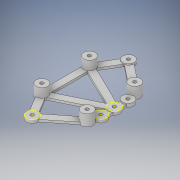
# Autodesk Inventor part: mount
Saved by Autodesk Inventor 2019 (Build 230136000, 136)
## iProperties
Created: 2019-01-14
Part Number: mount
Material: Generic
Document SubType Name: Modeling
Designer: erwin
Density: 1 g/cm^3
Appearance: Default
Author: erwin
Autodesk Inventor part; units mm, degrees
ref_plane "YZ Plane" through (0, 0, 0) normal (1, 0, 0) x (0, 1, 0)
ref_plane "XZ Plane" through (0, 0, 0) normal (0, 1, 0) x (-1, 0, 0)
ref_plane "XY Plane" through (0, 0, 0) normal (0, 0, 1) x (1, 0, 0)
sketch "Sketch1" plane through (0, 0, 0) normal (0, 1, 0) x (-1, 0, 0)
  point P0 (0, 0)
  point P1 (0, 0)
  point P2 (0, -12)
  point P3 (0, 12)
  point P4 (30, -42.5)
  point P5 (30, 42.5)
  dimension "d0" = 85
  dimension "d1" = 12
  dimension "d2" = 12
  dimension "d3" = 30
  dimension "d4" = 30.5
  dimension "d5" = 30.5
  constraints: 1 coincident
  measures "d0" distance of point (30, -42.5) point (30, 42.5)
  measures "d1" distance of point (0, 0) point (0, 12)
  measures "d2" distance of point (0, -12) point (0, 0)
  measures "d3" horizontal distance of point (30, 42.5) point (0, 12)
  measures "d4" vertical distance of point (0, 12) point (30, 42.5)
  measures "d5" vertical distance of point (0, -12) point (30, -42.5)
sketch "Sketch2" plane through (0, 0, 0) normal (0, 1, 0) x (-1, 0, 0)
  circle A0 centre (30, 42.5) radius 5
  point P0 (0, 0)
  dimension "d6" = 10
  constraints: 1 centre point, 1 coincident
  measures "d6" diameter of A0
extrude "Extrusion1" add sketch "Sketch2" along normal blind 3
sketch "Sketch3" plane through (-30, 3, 42.5) normal (0, 1, 0) x (1, 0, 0)
  circle A0 centre (0, 0) radius 5 projected
  point P0 (30, 42.5)
hole "Hole1" at (-30, 3, 42.5) direction (0, -1, 0) diameter 3 end through all both
pattern_sketch "Sketch Driven Pattern1" of "Extrusion1", "Hole1" from (-30, 0, 42.5) copies at (0, 0, 0) at (0, 0, -12) at (0, 0, 12) at (-30, 0, -42.5)
sketch "Sketch4" plane through (-30, 3, 42.5) normal (0, 1, 0) x (1, 0, 0)
  circle A0 centre (0, 0) radius 5 projected
  circle A1 centre (30, 30.5) radius 5 projected
  circle A2 centre (30, 42.5) radius 5 projected
  point P0 (30, 42.5)
sketch "Sketch5" plane through (0, 0, -12) normal (0, -1, 0) x (1, 0, 0)
  line L0 (-43, 33) -> (-3, 33) construction
  line L1 (-3, 33) -> (-3, -9) construction
  line L2 (-3, -9) -> (-43, -9) construction
  line L3 (-43, -9) -> (-43, 33) construction
  circle A0 centre (-30, 54.5) radius 1.5 construction
  circle A1 centre (-30, -30.5) radius 1.5 construction
  circle A2 centre (-43, 33) radius 5
  circle A3 centre (-43, -9) radius 5
  circle A4 centre (-3, -9) radius 5
  circle A5 centre (-3, 33) radius 5
  point P0 (0, 12)
  dimension "d16" = 40
  dimension "d17" = 42
  dimension "d18" = 3
  dimension "d19" = 21.5
  dimension "d20" = 21.5
  dimension "d21" = 10
  dimension "d22" = 10
  dimension "d23" = 10
  dimension "d24" = 10
  constraints: 8 end point, 4 centre point, 4 coincident, 2 parallel, 1 horizontal, 1 perpendicular
  measures "d16" distance of L1.end L2.end
  measures "d17" distance of L0.end L1.end
  measures "d18" distance from line of point (0, 12) L1
  measures "d19" distance from line of A0.centre L0
  measures "d20" distance from line of L2 A1.centre
  measures "d21" diameter of A2
  measures "d22" diameter of A3
  measures "d23" diameter of A4
  measures "d24" diameter of A5
extrude "Extrusion2" add sketch "Sketch5" against normal blind 10
sketch "Sketch7" plane through (-43, 10, 21) normal (0, 1, 0) x (1, 0, 0)
  circle A0 centre (0, 0) radius 5 projected
  circle A1 centre (0, 42) radius 5 projected
  circle A2 centre (40, 0) radius 5 projected
  circle A3 centre (40, 42) radius 5 projected
  point P0 (43, 21)
  constraints: 4 coincident
hole "Hole2" at (-43, 10, 21) at (-43, 10, -21) at (-3, 10, 21) at (-3, 10, -21) direction (0, -1, 0) diameter 3 end through all both
sketch "Sketch8" plane through (-30, 0, 42.5) normal (0, -1, 0) x (1, 0, 0)
  circle A0 centre (-13, -21.5) radius 1.5 projected
  circle A1 centre (-13, -21.5) radius 5 projected
  circle A2 centre (-13, -63.5) radius 1.5 projected
  circle A3 centre (-13, -63.5) radius 5 projected
  circle A4 centre (0, -85) radius 1.5 projected
  circle A5 centre (0, -85) radius 5 projected
  circle A6 centre (27, -21.5) radius 1.5 projected
  arc A7 (30, -25.5) -> (27, -26.5) centre (27, -21.5) ccw projected
  arc A8 (27, -26.5) -> (30, -25.5) centre (30, -30.5) ccw projected
  circle A9 centre (30, -30.5) radius 1.5 projected
  circle A10 centre (27, -63.5) radius 1.5 projected
  arc A11 (27, -58.5) -> (30, -59.5) centre (27, -63.5) ccw projected
  arc A12 (30, -59.5) -> (27, -58.5) centre (30, -54.5) ccw projected
  circle A13 centre (30, -54.5) radius 1.5 projected
  circle A14 centre (30, -42.5) radius 1.5 projected
  circle A15 centre (30, -42.5) radius 5 projected
  circle A16 centre (0, 0) radius 1.5 projected
  circle A17 centre (0, 0) radius 5 projected
  line L0 (0, 0) -> (-13, -21.5)
  line L1 (-13, -21.5) -> (-13, -63.5)
  line L2 (-13, -63.5) -> (0, -85)
  line L3 (0, -85) -> (27, -63.5)
  line L4 (0, 0) -> (27, -21.5)
  line L5 (30, -30.5) -> (30, -42.5)
  line L6 (30, -54.5) -> (30, -42.5)
  line L7 (0, 0) -> (-13, -21.5) construction
  line L8 (-4.6369, -1.8707) -> (-13.4975, -16.5248)
  arc A18 (2.5672, -1.5523) -> (-2.5672, 1.5523) centre (0, 0) ccw
  arc A19 (-15.5672, -19.9477) -> (-10.4328, -23.0523) centre (-13, -21.5) ccw
  line L9 (-13, -21.5) -> (-13, -63.5) construction
  line L10 (-16, -25.5) -> (-16, -59.5)
  arc A20 (-10, -21.5) -> (-16, -21.5) centre (-13, -21.5) ccw
  arc A21 (-16, -63.5) -> (-10, -63.5) centre (-13, -63.5) ccw
  line L11 (-13, -63.5) -> (0, -85) construction
  line L12 (-13.4975, -68.4752) -> (-4.6369, -83.1293)
  arc A22 (-10.4328, -61.9477) -> (-15.5672, -65.0523) centre (-13, -63.5) ccw
  arc A23 (-2.5672, -86.5523) -> (2.5672, -83.4477) centre (0, -85) ccw
  line L13 (0, -85) -> (27, -63.5) construction
  line L14 (4.9979, -84.8551) -> (25.7397, -68.3385)
  arc A24 (-1.8688, -82.6532) -> (1.8688, -87.3468) centre (0, -85) ccw
  arc A25 (28.8688, -65.8468) -> (25.1312, -61.1532) centre (27, -63.5) ccw
  line L15 (0, 0) -> (27, -21.5) construction
  line L16 (25.7397, -16.6615) -> (4.9979, -0.1449)
  arc A26 (1.8688, 2.3468) -> (-1.8688, -2.3468) centre (0, 0) ccw
  arc A27 (25.1312, -23.8468) -> (28.8688, -19.1532) centre (27, -21.5) ccw
  line L17 (30, -30.5) -> (30, -54.5) construction
  arc A28 (33, -30.5) -> (27, -30.5) centre (30, -30.5) ccw
  arc A29 (27, -54.5) -> (33, -54.5) centre (30, -54.5) ccw
  line L18 (33, -50.5) -> (33, -46.5)
  line L19 (33, -38.5) -> (33, -34.5)
  line L20 (27, -34.5) -> (27, -38.5)
  line L21 (27, -46.5) -> (27, -50.5)
  line L22 (22.0021, -63.6449) -> (1.2603, -80.1615)
  line L23 (-1.5652, -82.4114) -> (-1.8688, -82.6532)
  line L24 (2.5672, -83.4477) -> (2.3664, -83.1156)
  line L25 (0.4975, -80.0248) -> (-8.3631, -65.3707)
  line L26 (-10, -62.6635) -> (-10.4328, -61.9477)
  line L27 (-10, -63.5) -> (-10, -62.6635)
  line L28 (-10, -59.5) -> (-10, -25.5)
  line L29 (-10, -22.3365) -> (-10, -21.5)
  line L30 (-10.4328, -23.0523) -> (-10, -22.3365)
  line L31 (-8.3631, -19.6293) -> (0.4975, -4.9752)
  line L32 (2.3664, -1.8844) -> (2.5672, -1.5523)
  line L33 (-1.8688, -2.3468) -> (-1.5652, -2.5886)
  line L34 (1.2603, -4.8385) -> (22.0021, -21.3551)
  point P0 (30, -42.5)
  point P1 (-6.5, -10.75)
  point P2 (-13, -42.5)
  point P3 (-6.5, -74.25)
  point P4 (13.5, -74.25)
  point P5 (13.5, -10.75)
  dimension "d34" = 6
  dimension "d35" = 6
  dimension "d36" = 6
  dimension "d37" = 6
  dimension "d38" = 6
  dimension "d39" = 6
  constraints: 82 end point, 52 point on circle, 44 tangent, 20 parallel, 12 centre point, 6 midpoint, 4 collinear, 4 point on line, 3 vertical
  measures "d34" diameter of A19
  measures "d35" diameter of A21
  measures "d36" diameter of A23
  measures "d37" diameter of A25
  measures "d38" diameter of A27
  measures "d39" diameter of A29
extrude "Extrusion3" add sketch "Sketch8" against normal blind 2 contours L0 A17 L31 A1 | A1 L8 A17 L0 | L1 A3 L10 A1 | A1 L28 A3 L1 | A17 L4 A7 L34 | A3 L2 A5 L12 | A17 L16 A7 L4 | A3 L25 A5 L2 | A8 L5 A15 L20 | A5 L3 A11 L14 | L22 A11 L3 A5 | A8 L19 A15 L5 | A15 L6 A12 L21 | A15 L18 A12 L6
sketch "Sketch9" plane through (0, 0, 0) normal (0, -1, 0) x (1, 0, 0)
  circle A0 centre (0, 0) radius 1.5 projected
  circle A1 centre (-3, -21) radius 1.5 projected
  circle A2 centre (0, -12) radius 1.5 projected
  circle A3 centre (-30, 42.5) radius 1.5 projected
  circle A4 centre (-3, 21) radius 1.5 projected
  circle A5 centre (0, 12) radius 1.5 projected
  circle A6 centre (-30, -42.5) radius 1.5 projected
  line L0 (-40, 17) -> (-40, -17) projected
  arc A7 (-38.3631, -22.8707) -> (-40, -17) centre (-43, -21) ccw projected
  line L1 (-38.3631, -22.8707) -> (-29.5025, -37.5248) projected
  arc A8 (-28.7397, -37.6615) -> (-29.5025, -37.5248) centre (-30, -42.5) ccw projected
  line L2 (-28.7397, -37.6615) -> (-7.9979, -21.1449) projected
  arc A9 (-3, -16) -> (-7.9979, -21.1449) centre (-3, -21) ccw projected
  arc A10 (-3, -8) -> (-3, -16) centre (0, -12) ccw projected
  line L3 (-3, -8) -> (-3, -4) projected
  arc A11 (-3, 4) -> (-3, -4) centre (0, 0) ccw projected
  line L4 (-3, 4) -> (-3, 8) projected
  arc A12 (-3, 16) -> (-3, 8) centre (0, 12) ccw projected
  arc A13 (-7.9979, 21.1449) -> (-3, 16) centre (-3, 21) ccw projected
  line L5 (-7.9979, 21.1449) -> (-28.7397, 37.6615) projected
  arc A14 (-29.5025, 37.5248) -> (-28.7397, 37.6615) centre (-30, 42.5) ccw projected
  line L6 (-29.5025, 37.5248) -> (-38.3631, 22.8707) projected
  arc A15 (-40, 17) -> (-38.3631, 22.8707) centre (-43, 21) ccw projected
  line L7 (-46, -17) -> (-46, 17) projected
  arc A16 (-43.4975, 25.9752) -> (-46, 17) centre (-43, 21) ccw projected
  line L8 (-43.4975, 25.9752) -> (-34.6369, 40.6293) projected
  arc A17 (-25.0021, 42.3551) -> (-34.6369, 40.6293) centre (-30, 42.5) ccw projected
  line L9 (-25.0021, 42.3551) -> (-4.2603, 25.8385) projected
  arc A18 (0, 17) -> (-4.2603, 25.8385) centre (-3, 21) ccw projected
  arc A19 (3, 8) -> (0, 17) centre (0, 12) ccw projected
  line L10 (3, 8) -> (3, 4) projected
  arc A20 (3, -4) -> (3, 4) centre (0, 0) ccw projected
  line L11 (3, -4) -> (3, -8) projected
  arc A21 (0, -17) -> (3, -8) centre (0, -12) ccw projected
  arc A22 (-4.2603, -25.8385) -> (0, -17) centre (-3, -21) ccw projected
  line L12 (-4.2603, -25.8385) -> (-25.0021, -42.3551) projected
  arc A23 (-34.6369, -40.6293) -> (-25.0021, -42.3551) centre (-30, -42.5) ccw projected
  line L13 (-34.6369, -40.6293) -> (-43.4975, -25.9752) projected
  arc A24 (-46, -17) -> (-43.4975, -25.9752) centre (-43, -21) ccw projected
  circle A25 centre (-43, -21) radius 1.5 projected
  circle A26 centre (-43, 21) radius 1.5 projected
  line L14 (-3, 4.8038) -> (-38.0892, 21.9404)
  arc A27 (-41.6835, 23.6957) -> (-44.3165, 18.3043) centre (-43, 21) ccw
  arc A28 (-1.3165, -2.6957) -> (1.3165, 2.6957) centre (0, 0) ccw
  line L15 (-43, -21) -> (0, 0) construction
  line L16 (-38.0892, -21.9404) -> (-3, -4.8038)
  arc A29 (-44.3165, -18.3043) -> (-41.6835, -23.6957) centre (-43, -21) ccw
  arc A30 (1.3165, -2.6957) -> (-1.3165, 2.6957) centre (0, 0) ccw
  line L17 (-43, 21) -> (-3.4181, 1.6693) construction
  line L18 (-1.3479, 0.6583) -> (0, 0) construction
  line L19 (-1.3165, 2.6957) -> (-3.4181, 1.6693)
  line L20 (-6.8363, 0) -> (-40, -16.1962)
  line L21 (-40, 16.1962) -> (-6.8363, 0)
  line L22 (-3.4181, -1.6693) -> (-1.3165, -2.6957)
  point P0 (0, 0)
  point P1 (-21.5, 10.5)
  point P2 (-21.5, -10.5)
  dimension "d42" = 6
  dimension "d43" = 6
  constraints: 20 end point, 12 tangent, 10 point on circle, 6 point on line, 4 centre point, 4 parallel, 1 concentric, 1 midpoint, 2 other
  measures "d42" diameter of A28
  measures "d43" diameter of A30
extrude "Extrusion4" add sketch "Sketch9" against normal blind 2 contours A15 L14 L4 A11 L3 L16 A7 L0 L20 L21
equation "\"d2\" = d1"
equation "\"d5\" = d4"
equation "\"d20\" = d19"
body "Solid1"
